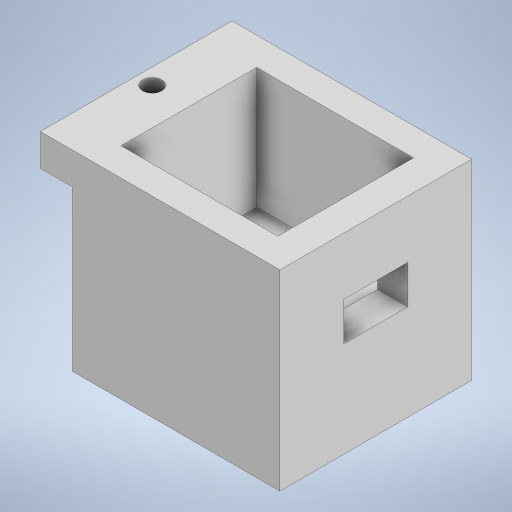
# Autodesk Inventor part: Top Sensor Mount
Saved by Autodesk Inventor 2023 (Build 270158000, 158)
## iProperties
Created: 2023-01-24
Part Number: Top Sensor Mount
Material: Generic
Document SubType Name: Modeling
Designer: Ahmed Nazir
Density: 1 g/cm^3
Appearance: Default
Author: Ahmed Nazir
Autodesk Inventor part; units mm, degrees
ref_plane "YZ Plane" through (0, 0, 0) normal (1, 0, 0) x (0, 1, 0)
ref_plane "XZ Plane" through (0, 0, 0) normal (0, 1, 0) x (-1, 0, 0)
ref_plane "XY Plane" through (0, 0, 0) normal (0, 0, 1) x (1, 0, 0)
sketch "Sketch1" plane through (0, 0, 0) normal (1, 0, 0) x (0, 1, 0)
  line L0 (0, 0) -> (30, 0)
  line L1 (30, 0) -> (30, -30)
  line L2 (30, -30) -> (0, -30)
  line L3 (0, -30) -> (0, 0)
  line L4 (0, -8.4131) -> (10, -3.75)
  line L5 (10, -3.75) -> (10, -26.25)
  line L6 (10, -26.25) -> (0, -21.5869)
  point P0 (10, -15)
  point P1 (0, -15)
  dimension "d0" = 30
  dimension "d1" = 30
  dimension "d2" = 10
  dimension "d3" = 22.5
  dimension "d4" = 65
  dimension "d5" = 65
  constraints: 14 end point, 2 midpoint, 2 parallel, 2 point on line, 1 horizontal, 1 horizontal alignment, 1 perpendicular, 1 vertical
  measures "d0" distance of L1.end L2.end
  measures "d1" distance of L0.end L1.end
  measures "d2" distance between parallel lines of L5 L3
  measures "d3" distance of L4.end L5.end
  measures "d4" angle of L3 L4
  measures "d5" angle of L3 L6
extrude "Extrusion1" add sketch "Sketch1" along normal blind 30 contours L0 L1 L2 L3 L6 L5 L4
sketch "Sketch2" plane through (30, 0, 0) normal (1, 0, 0) x (0, 0, -1)
  line L0 (0, 30) -> (0, 0) projected
  line L1 (21.5869, 0) -> (30, 0) projected
  line L2 (0, 30) -> (30, 30)
  line L3 (30, 30) -> (30, 0)
  line L4 (30, 0) -> (0, 0)
  line L5 (0, 0) -> (0, 30)
  point P0 (21.5869, 0)
  constraints: 8 end point, 2 parallel, 1 horizontal, 1 perpendicular
extrude "Extrusion2" add sketch "Sketch2" along normal blind 2.5
sketch "Sketch3" plane through (0, 0, 0) normal (-1, 0, 0) x (0, 0, 1)
  line L0 (-30, 0) -> (-30, 30) projected
  line L1 (0, 30) -> (0, 0) projected
  line L2 (-30, 30) -> (0, 30)
  line L3 (0, 30) -> (0, 25)
  line L4 (0, 25) -> (-30, 25)
  line L5 (-30, 25) -> (-30, 30)
  point P0 (0, 30)
  dimension "d10" = 5
  constraints: 8 end point, 2 parallel, 1 horizontal, 1 perpendicular, 1 point on line
  measures "d10" distance between parallel lines of L4 L2
extrude "Extrusion3" add sketch "Sketch3" along normal blind 5
sketch "Sketch4" plane through (32.5, 30, 0) normal (0, 1, 0) x (1, 0, 0)
  line L0 (-32.5, 0) -> (-37.5, 0) projected
  line L1 (-32.5, 0) -> (-32.5, 30) construction
  circle A0 centre (-35, 15) radius 1.5
  dimension "d13" = 3
  constraints: 2 end point, 1 centre point
  measures "d13" diameter of A0
extrude "Extrusion4" cut sketch "Sketch4" against normal through all
sketch "Sketch5" plane through (32.5, 30, 0) normal (0, 1, 0) x (1, 0, 0)
  line L0 (-29.2486, 25.6211) -> (-4.7242, 25.6211)
  line L1 (-4.7242, 25.6211) -> (-4.7242, 4.3789)
  line L2 (-4.7242, 4.3789) -> (-29.2486, 4.3789)
  line L3 (-29.2486, 4.3789) -> (-29.2486, 25.6211)
  line L4 (0, 30) -> (0, 0) projected
  point P0 (-32.5, 0)
  point P1 (0, 15)
  point P2 (-4.7242, 15)
  point P3 (0, 15)
  constraints: 8 end point, 3 midpoint, 2 parallel, 1 horizontal, 1 horizontal alignment, 1 perpendicular
extrude "Extrusion5" cut sketch "Sketch5" against normal blind 19
sketch "Sketch6" plane through (32.5, 0, 0) normal (1, 0, 0) x (0, 0, -1)
  line L0 (25.6211, 11) -> (4.3789, 11) projected
  line L1 (10, 21) -> (20, 21)
  line L2 (20, 21) -> (20, 15)
  line L3 (20, 15) -> (10, 15)
  line L4 (10, 15) -> (10, 21)
  point P0 (0, 0)
  point P1 (15, 15)
  point P2 (15, 11)
  dimension "d18" = 10
  dimension "d19" = 6
  dimension "d20" = 4
  constraints: 8 end point, 2 midpoint, 2 parallel, 1 horizontal, 1 perpendicular, 1 vertical alignment
  measures "d18" distance of L2.end L3.end
  measures "d19" distance of L1.end L2.end
  measures "d20" distance between parallel lines of L3 L0
extrude "Extrusion6" cut sketch "Sketch6" against normal up to next
body "Solid1"
